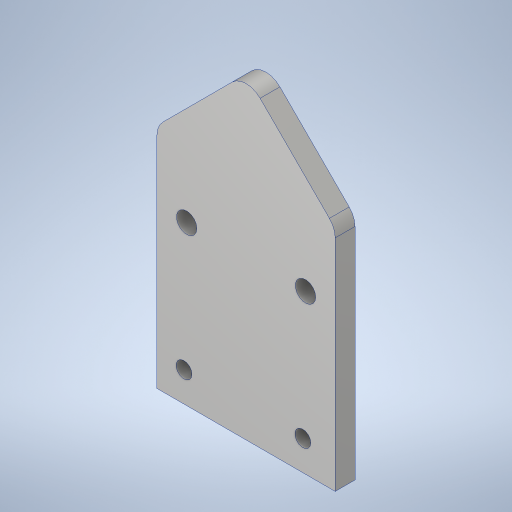
# Autodesk Inventor part: CL7-005
Saved by Autodesk Inventor 2023.4 (Build 274418000, 418)
## iProperties
Created: 2025-03-17
Part Number: CL7-005
Material: Aluminum 6061
Document SubType Name: Modeling
Designer: dlangdon
Density: 2.7 g/cm^3
Appearance: Aluminum - Flat
Author: dlangdon
Autodesk Inventor part; units mm, degrees
ref_plane "YZ Plane" through (0, 0, 0) normal (1, 0, 0) x (0, 1, 0)
ref_plane "XZ Plane" through (0, 0, 0) normal (0, 1, 0) x (-1, 0, 0)
ref_plane "XY Plane" through (0, 0, 0) normal (0, 0, 1) x (1, 0, 0)
sketch "Sketch1" plane through (0, 0, 0) normal (0, 0, 1) x (1, 0, 0)
  line L0 (-19.05, 0) -> (19.05, 0) construction
  circle A0 centre (-19.05, 0) radius 3.2639
  circle A1 centre (19.05, 0) radius 3.2639
  line L1 (-28.575, 19.5947) -> (-28.575, -50.8)
  line L2 (-28.575, -50.8) -> (28.575, -50.8)
  line L3 (28.575, -50.8) -> (28.575, 19.5947)
  line L4 (-26.7151, 24.0849) -> (-4.4901, 46.3099)
  line L5 (4.4901, 46.3099) -> (26.7151, 24.0849)
  arc A2 (4.4901, 46.3099) -> (-4.4901, 46.3099) centre (0, 41.8197) ccw
  arc A3 (-26.7151, 24.0849) -> (-28.575, 19.5947) centre (-22.225, 19.5947) ccw
  arc A4 (28.575, 19.5947) -> (26.7151, 24.0849) centre (22.225, 19.5947) ccw
  point P0 (0, 0)
  point P1 (0, 0)
  point P2 (0, 50.8)
  point P3 (28.575, 22.225)
  point P4 (-28.575, 22.225)
  point P5 (0, -50.8)
  dimension "d0" = 6.5278
  dimension "d1" = 38.1
  dimension "d4" = 50.8
  dimension "d17" = 101.6
  dimension "d18" = 57.15
  dimension "d19" = 6.35
  constraints: 12 end point, 6 point on circle, 6 point on line, 6 tangent, 5 centre point, 3 coincident, 3 equal radius, 2 midpoint, 2 perpendicular, 2 vertical, 2 vertical alignment, 1 horizontal, 1 horizontal alignment
  measures "d0" diameter of A0
  measures "d1" distance of L0.start L0.end
  measures "d4" distance from line of A1.centre L2
  measures "d17" distance from line of L2 point (0, 50.8)
  measures "d18" distance of L1.end L2.end
  measures "d19" radius of A2
extrude "Extrusion1" add sketch "Sketch1" along normal blind 6.35
sketch "Sketch2" plane through (0, 0, 6.35) normal (0, 0, 1) x (1, 0, 0)
  line L0 (-19.9009, -41.275) -> (18.1991, -41.275) construction
  line L1 (-28.575, -50.8) -> (28.575, -50.8) projected
  point P0 (0, 0)
  dimension "d8" = 38.1
  dimension "d9" = 9.525
  constraints: 2 coincident, 2 end point, 1 horizontal
  measures "d8" distance of L0.start L0.end
  measures "d9" distance between parallel lines of L0 L1
hole "Hole1" at (-19.9009, -41.275, 6.35) at (18.1991, -41.275, 6.35) direction (0, 0, -1) diameter 5.1054 end through all clearance for "Flat Head Machine Screw (82)" size "#10" standard "Ansi Unified Screw Threads"
body "Solid1"
